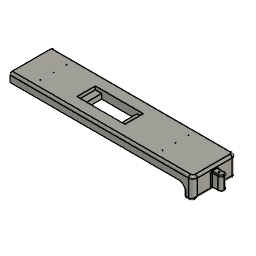
Timon (Autodesk Fusion 360 design; units mm, degrees)
Autodesk Fusion 360 part; units mm, degrees
sketch "Boceto1" plane through (0, 0, 0) normal (0, 0, 1) x (1, 0, 0)
  line L0 (0, 0) -> (-200, 0)
  line L1 (-200, 0) -> (-200, 50)
  line L2 (-200, 50) -> (0, 50)
  line L3 (0, 50) -> (0, 0)
  dimension "d1" = 200
  dimension "d2" = 50
  constraint horizontal L0
  constraint vertical L1
  constraint horizontal L2
  constraint vertical L3
  constraint coincident L0.start L3.end
  measures "d1" distance of L0.start L0.end
  measures "d2" distance of L0.start L2.end
extrude "Extruir1" add sketch "Boceto1" along normal blind 20
sketch "Boceto2" plane through (0, 0, 0) normal (1, 0, 0) x (0, 1, 0)
  line L0 (0, 0) -> (50, 0)
  line L1 (50, 0) -> (50, 20)
  line L2 (50, 20) -> (0, 20)
  line L3 (0, 20) -> (0, 0)
  line L4 (0, 20) -> (50, 20)
  line L5 (50, 20) -> (50, -15)
  line L6 (50, -15) -> (0, -15)
  line L7 (0, -15) -> (0, 20)
  line L8 (25, 20) -> (25, -15)
  line L9 (21.215, -10) -> (28.785, -10)
  line L10 (21.215, -10) -> (28.785, -10)
  line L11 (28.785, -10) -> (28.785, 6)
  line L12 (28.785, 6) -> (21.215, 6)
  line L13 (21.215, 6) -> (21.215, -10)
  line L14 (25, -15) -> (25, -10)
  line L15 (25, -10) -> (28.785, -10)
  dimension "d5" = 35
  dimension "d7" = 7.57
  dimension "d8" = 16
  dimension "d30" = 5
  constraint horizontal L4
  constraint vertical L5
  constraint horizontal L6
  constraint vertical L7
  constraint coincident L2.end L3.start
  constraint midpoint L2 L8.start
  constraint midpoint L6 L8.end
  constraint perpendicular L6 L8
  constraint perpendicular L8 L9
  constraint perpendicular L10 L11
  constraint parallel L10 L12
  constraint parallel L11 L13
  constraint perpendicular L9 L14
  constraint perpendicular L11 L15
  measures "d5" distance of L2.end L6.end
  measures "d7" distance of L9.start L9.end
  measures "d8" distance of L9.start L12.end
  measures "d30" distance of L8.end L14.end
extrude "Extruir2" add sketch "Boceto2" along normal blind 10
extrude "Extruir3" add sketch "Boceto2" along normal blind 21 contours L0 L8 L12 L13 | L0 L8 L9 L10 L13 | L0 L8 L11 L12 | L0 L8 L9 L10 L11 L15
sketch "Boceto3" plane through (0, 0, 6) normal (0, 0, 1) x (-1, 0, 0)
  line L0 (-10, -28.785) -> (-10, -21.215)
  line L1 (-10, -21.215) -> (-21, -21.215)
  line L2 (-21, -21.215) -> (-21, -28.785)
  line L3 (-21, -28.785) -> (-10, -28.785)
  line L4 (-10, -25) -> (-14.22, -25)
  circle A0 centre (-15.07, -25) radius 0.85
  dimension "d13" = 4.22
  dimension "d14" = 1.7
  constraint midpoint L0 L4.start
  constraint perpendicular L0 L4
  constraint coincident L4.end A0
  measures "d13" distance of L4.start L4.end
  measures "d14" diameter of A0
extrude "Extruir4" cut sketch "Boceto3" against normal blind 22 contours A0
fillet "Empalme1" radius 3.5 2 edges at (21, 28.785, -2) (21, 21.215, -2)
fillet "Empalme2" radius 5 4 edges at (10, 0, 2.5) (10, 25, 20) (10, 50, 2.5) (10, 25, -15)
ref_plane "PlanoDeObra1" through (-95, 25, 2.5) normal (0, -1, 0) x (1, 0, 0)
sketch "Boceto4" plane through (0, 25, 0) normal (0, -1, 0) x (-1, 0, 0)
sketch "Boceto5" plane through (0, 0, 0) normal (0, 0, -1) x (1, 0, 0)
  line L0 (-200, -50) -> (0, -50)
  line L1 (0, -50) -> (0, 0)
  line L2 (0, 0) -> (-200, 0)
  line L3 (-200, 0) -> (-200, -50)
  line L4 (-10, -25) -> (0, 0)
  line L5 (-10, -25) -> (0, -50)
  line L6 (0, 0) -> (0, -50)
  constraint coincident L1.end L2.start
  constraint coincident L0.end L1.start
extrude "Extruir5" add sketch "Boceto5" along normal blind 15 contours L1 L4 L5 L6
fillet "Empalme3" radius 2.5 8 edges at (-5, 12.5, -15) (0, 0, -7.5) (-5, 37.5, -15) (0, 50, -7.5) (2.5, 50, -15) (8.5355, 48.5355, -13.5355) (2.5, 0, -15) (8.5355, 1.4645, -13.5355)
fillet "Empalme4" radius 6 4 edges at (0.291, 49.5702, 0) (-5.3143, 36.7142, 0) (-5.3143, 13.2858, 0) (0.291, 0.4298, 0)
fillet "Empalme5" radius 1 12 edges at (13.75, 21.215, -10) (19.9749, 22.2401, -10) (21, 25, -10) (19.9749, 27.7599, -10) (13.75, 28.785, -10) (13.75, 21.215, 6) (19.9749, 22.2401, 6) (21, 25, 6) (19.9749, 27.7599, 6) (13.75, 28.785, 6) (10, 28.785, -2) (10, 21.215, -2)
sketch "Boceto6" plane through (0, 0, 20) normal (0, 0, 1) x (-1, 0, 0)
  line L0 (-5, 0) -> (-5, -50)
  line L1 (-5, -50) -> (200, -50)
  line L2 (200, -50) -> (200, 0)
  line L3 (200, 0) -> (-5, 0)
  line L4 (110, -50) -> (110, 0)
  line L5 (82.5, -14.5) -> (137.5, -14.5)
  line L6 (137.5, -14.5) -> (137.5, -35.5)
  line L7 (137.5, -35.5) -> (82.5, -35.5)
  line L8 (82.5, -35.5) -> (82.5, -14.5)
  line L9 (82.5, -14.5) -> (137.5, -35.5) construction
  line L10 (137.5, -14.5) -> (82.5, -35.5) construction
  line L11 (89.75, -14.5) -> (130.25, -14.5)
  line L12 (130.25, -14.5) -> (130.25, -35.5)
  line L13 (130.25, -35.5) -> (89.75, -35.5)
  line L14 (89.75, -35.5) -> (89.75, -14.5)
  line L15 (89.75, -14.5) -> (130.25, -35.5) construction
  line L16 (130.25, -14.5) -> (89.75, -35.5) construction
  point P0 (110, -25)
  point P1 (110, -25)
  dimension "d31" = 55
  dimension "d32" = 21
  dimension "d33" = 40.5
  dimension "d34" = 21
  constraint coincident L1 L4.start
  constraint coincident L3 L4.end
  constraint perpendicular L3 L4
  constraint horizontal L5
  constraint perpendicular L5 L6
  constraint parallel L5 L7
  constraint parallel L6 L8
  constraint coincident L9 P1
  constraint coincident L10 P1
  constraint midpoint L4 P1
  constraint horizontal L11
  constraint perpendicular L11 L12
  constraint parallel L11 L13
  constraint parallel L12 L14
  constraint coincident L15 P1
  constraint coincident L16 P1
  constraint coincident P1 P0
  measures "d31" distance of L6.end L7.end
  measures "d32" distance of L5.end L6.end
  measures "d33" distance of L12.end L13.end
  measures "d34" distance of L11.end L12.end
extrude "Extruir6" cut sketch "Boceto6" against normal blind 40 contours L4 L5 L7 L11 L12 L13 | L4 L5 L7 L11 L13 L14
extrude "Extruir7" cut sketch "Boceto6" against normal blind 13.8 contours L5 L7 L8 L14 | L5 L6 L7 L12
extrude "Extruir8" cut 1 faces at (-24.166, 21.5, 20) along direction (0, 0, -1) blind 10
extrude "Extruir9" cut 1 faces at (5.001, 16.6667, 16.6667) along direction (1, 0, 0) blind 15
fillet "Empalme7" radius 0.5 4 edges at (-89.75, 25, 0) (-110, 35.5, 0) (-110, 14.5, 0) (-130.25, 25, 0)
fillet "Empalme8" radius 2.5 5 edges at (-97.5, 50, 10) (8.5355, 48.5355, 10) (10, 25, 10) (8.5355, 1.4645, 10) (-97.5, 0, 10)
sketch "Boceto7" plane through (0, 0, 10) normal (0, 0, 1) x (-1, 0, 0)
  line L0 (200, -2.5) -> (-5, -2.5)
  arc A0 (-5, -2.5) -> (-7.5, -5) centre (-5, -5) ccw
  line L1 (-7.5, -5) -> (-7.5, -45)
  arc A1 (-7.5, -45) -> (-5, -47.5) centre (-5, -45) ccw
  line L2 (-5, -47.5) -> (200, -47.5)
  line L3 (200, -47.5) -> (200, -2.5)
  line L4 (137.5, -35.5) -> (82.5, -35.5)
  line L5 (82.5, -35.5) -> (82.5, -14.5)
  line L6 (82.5, -14.5) -> (137.5, -14.5)
  line L7 (137.5, -14.5) -> (137.5, -35.5)
  circle A2 centre (175, -10) radius 0.5
  circle A3 centre (35, -10) radius 0.5
  circle A4 centre (175, -25) radius 0.5
  circle A5 centre (35, -25) radius 0.5
  circle A6 centre (175, -40) radius 0.5
  circle A7 centre (35, -40) radius 0.5
  point P0 (35, -10)
  point P1 (175, -25)
  point P2 (35, -25)
  point P3 (175, -40)
  point P4 (35, -40)
  dimension "d49" = 1
  dimension "d53" = -140
  dimension "d54" = -30
  dimension "d57" = -140
  dimension "d58" = -30
  measures "d49" diameter of A2
extrude "Extruir10" cut sketch "Boceto7" against normal blind 20 contours A2 | A3 | A4 | A5 | A6 | A7
